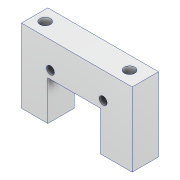
# Autodesk Inventor part: Espaciador Izquierdo
Saved by Autodesk Inventor 2020 (Build 240168000, 168)
## iProperties
Created: 2020-05-16
Part Number: Espaciador Izquierdo
Material: Aluminum 6061
Document SubType Name: Modeling
Designer: Dante
Density: 2.7 g/cm^3
Appearance: Aluminum - Flat
Mass: 21.752 g
Surface Area: 41.0545 cm^2
Volume: 8.05628 cm^3
Author: Dante
Autodesk Inventor part; units mm, degrees
ref_plane "YZ Plane" through (0, 0, 0) normal (1, 0, 0) x (0, 1, 0)
ref_plane "XZ Plane" through (0, 0, 0) normal (0, 1, 0) x (-1, 0, 0)
ref_plane "XY Plane" through (0, 0, 0) normal (0, 0, 1) x (1, 0, 0)
sketch "Sketch1" plane through (0, 0, 0) normal (0, 0, 1) x (1, 0, 0)
  line L0 (50, -5) -> (50, 23)
  line L1 (50, 23) -> (8, 23)
  line L2 (18, 10) -> (38, 10)
  line L3 (18, 10) -> (18, -5)
  line L4 (38, 10) -> (38, -5)
  line L5 (8, -5) -> (8, 23)
  line L6 (8, -5) -> (18, -5)
  line L7 (38, -5) -> (50, -5)
  dimension "d1" = 28
  dimension "d4" = 15
  dimension "d14" = 20
  dimension "d16" = 12
  dimension "d37" = 42
  dimension "d46" = 28
  constraints: 16 end point, 3 vertical, 2 horizontal, 1 collinear, 1 perpendicular
  measures "d1" distance of L0.start L0.end
  measures "d4" distance of L2.start L3.end
  measures "d14" distance of L2.start L2.end
  measures "d16" distance between parallel lines of L0 L4
  measures "d37" distance between parallel lines of L5 L0
  measures "d46" distance of L5.start L1.end
extrude "Extrusion3" add sketch "Sketch1" along normal blind 10
sketch "Sketch5" plane through (8, -5, 0) normal (0, -1, 0) x (1, 0, 0)
  circle A0 centre (4, 5) radius 2
  line L0 (10, 0) -> (10, 10) projected
  line L1 (0, 0) -> (10, 0) projected
  circle A1 centre (36, 5) radius 2
  line L2 (30, 0) -> (30, 10) projected
  line L3 (30, 0) -> (42, 0) projected
  dimension "d38" = 4
  dimension "d39" = 6
  dimension "d40" = 5
  dimension "d41" = 4
  dimension "d42" = 6
  dimension "d43" = 5
  constraints: 2 centre point
  measures "d38" diameter of A0
  measures "d39" distance from line of A0.centre L0
  measures "d40" distance from line of A0.centre L1
  measures "d41" diameter of A1
  measures "d42" distance from line of L2 A1.centre
  measures "d43" distance from line of L3 A1.centre
extrude "Extrusion6" cut sketch "Sketch5" against normal blind 100
sketch "Boceto6" plane through (0, 0, 10) normal (0, 0, 1) x (1, 0, 0)
  line L0 (50, 23) -> (8, 23) projected
  circle A0 centre (19, 13) radius 1.5
  circle A1 centre (39, 13) radius 1.5
  point P0 (0, 0)
  dimension "d50" = 3
  dimension "d51" = 3
  dimension "d52" = 10
  dimension "d53" = 10
  dimension "d54" = 20
  constraints: 2 centre point
  measures "d50" diameter of A0
  measures "d51" diameter of A1
  measures "d52" distance from line of L0 A0.centre
  measures "d53" distance from line of L0 A1.centre
  measures "d54" distance of A1.centre A0.centre
extrude "Extrusión7" cut sketch "Boceto6" against normal blind 10
thread "Rosca1" size "M3x0.5" class "6H" standard "ANSI Metric M Profile" length 12
thread "Rosca2" size "M3x0.5" class "6H" standard "ANSI Metric M Profile" length 12
body "Solid1"
